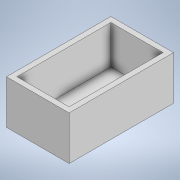
# Autodesk Inventor part: paraBox
Saved by Autodesk Inventor 2020 (Build 240168000, 168)
## iProperties
RuleStatus: InUse
Created: 2020-02-28
Part Number: paraBox
Material: Generic
Document SubType Name: Modeling
Designer: Eric
Density: 1 g/cm^3
Appearance: Default
Author: Eric
Autodesk Inventor part; units mm, degrees
ref_plane "YZ Plane" through (0, 0, 0) normal (1, 0, 0) x (0, 1, 0)
ref_plane "XZ Plane" through (0, 0, 0) normal (0, 1, 0) x (-1, 0, 0)
ref_plane "XY Plane" through (0, 0, 0) normal (0, 0, 1) x (1, 0, 0)
sketch "Sketch1" plane through (0, 0, 0) normal (0, 1, 0) x (-1, 0, 0)
  line L0 (0, 0) -> (76.2, 0)
  line L1 (76.2, 0) -> (76.2, -127)
  line L2 (76.2, -127) -> (0, -127)
  line L3 (0, -127) -> (0, 0)
  dimension "d0" = 76.2
  dimension "d1" = 127
  constraints: 8 end point, 2 parallel, 1 horizontal, 1 perpendicular
  measures "d0" distance of L1.end L2.end
  measures "d1" distance of L0.end L1.end
extrude "Extrusion1" add sketch "Sketch1" along normal blind 53.34
shell "Shell1" thickness 6.35 removed faces 1 at (-50.8, 53.34, -84.6667)
equation "\"d0\" = width"
equation "\"d1\" = length"
equation "\"d2\" = height"
equation "\"d4\" = material"
equation "\"length\" = 127"
equation "\"width\" = 76.2"
equation "\"height\" = 53.34"
equation "\"material\" = 6.35"
body "Solid1"
